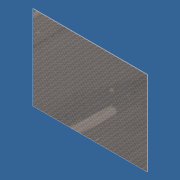
# Autodesk Inventor part: GE-11041-01
Saved by Autodesk Inventor 2012 (Build 160160000, 160)
## iProperties
Created: 2010-09-30
Part Number: GE-11041-01
Document SubType Name: Modeling
Designer: mcyr
Density: 1 g/cm^3
Description: Main Plate
Material: Default
Title: Main Plate
Author: mcyr
Autodesk Inventor part; units mm, degrees
ref_plane "YZ Plane" through (0, 0, 0) normal (1, 0, 0) x (0, 1, 0)
ref_plane "XZ Plane" through (0, 0, 0) normal (0, 1, 0) x (-1, 0, 0)
ref_plane "XY Plane" through (0, 0, 0) normal (0, 0, 1) x (1, 0, 0)
sketch "Sketch1" plane through (0, 0, 0) normal (0, 0, 1) x (1, 0, 0)
  line L0 (-25.5063, 25.217) -> (1212.7437, 25.217)
  line L1 (1212.7437, 25.217) -> (1212.7437, -889.183)
  line L2 (1212.7437, -889.183) -> (-25.5063, -889.183)
  line L3 (-25.5063, -889.183) -> (-25.5063, 25.217)
  point P0 (0, 0)
  dimension "d0" = 1238.25
  dimension "d1" = 914.4
  constraints: 8 end point, 2 parallel, 1 horizontal, 1 perpendicular
  measures "d0" distance of L0.start L0.end
  measures "d1" distance of L2.end L0.start
extrude "Extrusion1" add sketch "Sketch1" along normal blind 4.7625
body "Solid1"
